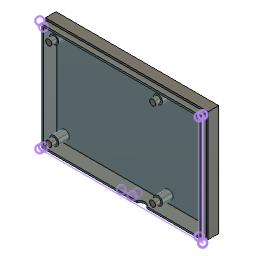
bottom-enclosure-v1 (Autodesk Fusion 360 design; units mm, degrees)
part number: 2026-06-12-23-29-13-626
Autodesk Fusion 360 part; units mm, degrees
note: some values were not read from the file. Set by a fixed rule: which sketch regions a step uses.
sketch "Sketch1" plane through (0, 0, 0) normal (0, 0, 1) x (1, 0, 0)
sketch "Sketch2" plane through (0, 0, 0) normal (0, 0, 1) x (1, 0, 0)
  line L0 (44.5, 30) -> (-44.5, 30)
  line L1 (-44.5, 30) -> (-44.5, -30)
  line L2 (-44.5, -30) -> (44.5, -30)
  line L3 (44.5, -30) -> (44.5, 30)
  line L4 (44.5, 30) -> (-44.5, -30) construction
  line L5 (-44.5, 30) -> (44.5, -30) construction
  dimension "d1" = 89
  dimension "d2" = 60
  constraint horizontal L0
  constraint perpendicular L0 L1
  constraint parallel L0 L2
  constraint parallel L1 L3
  constraint coincident L4 origin
  constraint coincident L5 origin
  measures "d1" distance of L1.end L2.end
  measures "d2" distance of L0.end L1.end
extrude "Extrude1" add sketch "Sketch2" along normal blind 1.5 makes body 1
sketch "Sketch3" plane through (0, 0, 1.5) normal (0, 0, 1) x (1, 0, 0)
  line L0 (44.5, -30) -> (44.5, 30)
  line L1 (44.5, 30) -> (-44.5, 30)
  line L2 (-44.5, 30) -> (-44.5, -30)
  line L3 (-44.5, -30) -> (44.5, -30)
  line L4 (42.5, 28) -> (-42.5, 28)
  line L5 (-42.5, 28) -> (-42.5, -28)
  line L6 (-42.5, -28) -> (42.5, -28)
  line L7 (42.5, -28) -> (42.5, 28)
  line L8 (42.5, 28) -> (-42.5, -28) construction
  line L9 (-42.5, 28) -> (42.5, -28) construction
  line L10 (44.5, 30) -> (-44.5, 30)
  line L11 (-44.5, 30) -> (-44.5, -30)
  line L12 (-44.5, -30) -> (44.5, -30)
  line L13 (44.5, -30) -> (44.5, 30)
  line L14 (44.5, 30) -> (-44.5, -30) construction
  line L15 (-44.5, 30) -> (44.5, -30) construction
  dimension "d5" = 85
  dimension "d6" = 56
  dimension "d7" = 89
  dimension "d8" = 60
  constraint horizontal L4
  constraint perpendicular L4 L5
  constraint parallel L4 L6
  constraint parallel L5 L7
  constraint coincident L8 origin
  constraint coincident L9 origin
  constraint horizontal L10
  constraint perpendicular L10 L11
  constraint parallel L10 L12
  constraint parallel L11 L13
  constraint coincident L14 origin
  constraint coincident L15 origin
  measures "d5" distance of L5.end L6.end
  measures "d6" distance of L4.end L5.end
  measures "d7" distance of L2.end L0.start
  measures "d8" distance of L1.end L2.end
extrude "Extrude2" add sketch "Sketch3" along normal blind 7.5 bodies 1
sketch "Sketch4" plane through (0, 0, 1.5) normal (0, 0, 1) x (1, 0, 0)
  line L0 (42.5, 28) -> (-42.5, 28)
  line L1 (-42.5, 28) -> (-42.5, -28)
  line L2 (-42.5, -28) -> (42.5, -28)
  line L3 (42.5, -28) -> (42.5, 28)
  circle A0 centre (-39, 24.5) radius 2.5
  circle A1 centre (-39, -24.5) radius 2.5
  circle A2 centre (19, 24.5) radius 2.5
  circle A3 centre (19, -24.5) radius 2.5
  dimension "d11" = 85
  dimension "d12" = 56
  dimension "d13" = 5
  dimension "d14" = 5
  dimension "d15" = 5
  dimension "d16" = 5
  dimension "d17" = 49
  dimension "d18" = 58
  dimension "d19" = 3.5
  dimension "d20" = 3.5
  constraint horizontal A0.centre A2.centre
  constraint horizontal A1.centre A3.centre
  constraint vertical A2.centre A3.centre
  measures "d11" distance of L1 L3
  measures "d12" distance of L0 L2
  measures "d13" diameter of A0
  measures "d14" diameter of A1
  measures "d15" diameter of A2
  measures "d16" diameter of A3
  measures "d17" distance of A0.centre A1.centre
  measures "d18" distance of A0.centre A2.centre
  measures "d19" distance of L0 A0.centre
  measures "d20" distance of L1 A1.centre
extrude "Extrude3" add sketch "Sketch4" along normal blind 6 contours A0 | A1 | A2 | A3 bodies 1
sketch "Sketch5" plane through (0, 0, 7.5) normal (0, 0, 1) x (1, 0, 0)
  circle A0 centre (-39, 24.5) radius 2.5
  circle A1 centre (-39, 24.5) radius 1.65
  circle A2 centre (-39, -24.5) radius 1.65
  circle A3 centre (19, -24.5) radius 1.65
  circle A4 centre (19, 24.5) radius 1.65
  dimension "d23" = 3.3
  dimension "d24" = 3.3
  dimension "d25" = 3.3
  dimension "d26" = 3.3
  constraint concentric A0 A1
  measures "d23" diameter of A1
  measures "d24" diameter of A2
  measures "d25" diameter of A3
  measures "d26" diameter of A4
extrude "Extrude4" add sketch "Sketch5" along normal blind 3 contours A1 | A2 | A3 | A4 bodies 1
sketch "Sketch6" plane through (0, 0, 1.5) normal (0, 0, 1) x (1, 0, 0)
  circle A0 centre (-39, -24.5) radius 2.5
  circle A1 centre (-39, 24.5) radius 2.5
  circle A2 centre (19, -24.5) radius 2.5
  circle A3 centre (19, 24.5) radius 2.5
  line L0 (42.5, 28) -> (-42.5, 28)
  line L1 (-42.5, 28) -> (-42.5, -28)
  line L2 (-42.5, -28) -> (42.5, -28)
  line L3 (42.5, -28) -> (42.5, 28)
sketch "Sketch7" plane through (0, 0, 9) normal (0, 0, 1) x (1, 0, 0)
  line L0 (42.5, 28) -> (42.5, -28)
  line L1 (42.5, -28) -> (-42.5, -28)
  line L2 (-42.5, -28) -> (-42.5, 28)
  line L3 (-42.5, 28) -> (42.5, 28)
  line L4 (44.5, -30) -> (44.5, 30)
  line L5 (44.5, 30) -> (-44.5, 30)
  line L6 (-44.5, 30) -> (-44.5, -30)
  line L7 (-44.5, -30) -> (44.5, -30)
  line L8 (0, 30) -> (5, 30)
  line L9 (5, 30) -> (5, 32)
  line L10 (5, 32) -> (0, 32)
  line L11 (0, 32) -> (0, 30)
  line L12 (0, 30) -> (-5, 30)
  line L13 (-5, 30) -> (-5, 32)
  line L14 (-5, 32) -> (0, 32)
  line L15 (0, 32) -> (0, 30)
  line L16 (0, -30) -> (5, -30)
  line L17 (5, -30) -> (5, -32)
  line L18 (5, -32) -> (0, -32)
  line L19 (0, -32) -> (0, -30)
  line L20 (0, -30) -> (-5, -30)
  line L21 (-5, -30) -> (-5, -32)
  line L22 (-5, -32) -> (0, -32)
  line L23 (0, -32) -> (0, -30)
  dimension "d29" = 5
  dimension "d30" = 2
  dimension "d31" = 2
  dimension "d32" = 5
  dimension "d33" = 2
  dimension "d34" = 5
  constraint horizontal L8
  constraint vertical L9
  constraint horizontal L10
  constraint vertical L11
  constraint midpoint L5 L8.start
  constraint horizontal L12
  constraint vertical L13
  constraint horizontal L14
  constraint vertical L15
  constraint horizontal L16
  constraint vertical L17
  constraint horizontal L18
  constraint vertical L19
  constraint midpoint L7 L16.start
  constraint horizontal L20
  constraint vertical L21
  constraint horizontal L22
  constraint vertical L23
  measures "d29" distance of L8.start L8.end
  measures "d30" distance of L8.start L10.end
  measures "d31" distance of L8.start L10.end
  measures "d32" distance of L16.start L16.end
  measures "d33" distance of L16.start L18.end
  measures "d34" distance of L16.start L20.end
extrude "Extrude5" add sketch "Sketch7" against normal blind 4 contours L7 L16 L17 L18 L19 L23 | L5 L8 L9 L10 L11 L15 | L7 L19 L20 L21 L22 L23 | L5 L11 L12 L13 L14 L15 bodies 1
extrude "Extrude6" add 2 faces at (-1.6667, -30.6667, 5) (-1.6667, 31.3333, 5) along direction (0, 0, -1) blind 4 on bodies 1 bodies 1
extrude "Extrude7" add 2 faces at (-1.6667, 31.3333, 1) (-1.6667, -30.6667, 1) along direction (0, 0, -1) blind 1 on bodies 1 bodies 1
sketch "Sketch8" plane through (0, 0, 9) normal (0, 0, 1) x (1, 0, 0)
  line L0 (42.5, 28) -> (42.5, -28)
  line L1 (42.5, -28) -> (-42.5, -28)
  line L2 (-42.5, -28) -> (-42.5, 28)
  line L3 (-42.5, 28) -> (42.5, 28)
  line L4 (44.5, -30) -> (44.5, 30)
  line L5 (44.5, 30) -> (5, 30)
  line L6 (5, 30) -> (5, 32)
  line L7 (5, 32) -> (-5, 32)
  line L8 (-5, 32) -> (-5, 30)
  line L9 (-5, 30) -> (-44.5, 30)
  line L10 (-44.5, 30) -> (-44.5, -30)
  line L11 (-44.5, -30) -> (-5, -30)
  line L12 (-5, -30) -> (-5, -32)
  line L13 (-5, -32) -> (5, -32)
  line L14 (5, -32) -> (5, -30)
  line L15 (5, -30) -> (44.5, -30)
  line L16 (5, -32) -> (-5, -32)
  line L17 (-5, -32) -> (-5, -30)
  line L18 (-5, -30) -> (5, -30)
  line L19 (5, -30) -> (5, -32)
  line L20 (5, 30) -> (-5, 30)
  line L21 (-5, 30) -> (-5, 32)
  line L22 (-5, 32) -> (5, 32)
  line L23 (5, 32) -> (5, 30)
  constraint horizontal L16
  constraint vertical L17
  constraint horizontal L18
  constraint vertical L19
  constraint coincident L11.end L12.start
  constraint coincident L13.end L14.start
  constraint horizontal L20
  constraint vertical L21
  constraint horizontal L22
  constraint vertical L23
  constraint coincident L7.end L8.start
  constraint coincident L5.end L6.start
extrude "Extrude8" cut sketch "Sketch8" against normal blind 2 contours L12 L13 L14 L16 L17 L18 L19 | L6 L7 L8 L20 L21 L22 L23 bodies 1
fillet "Fillet1" radius 1 1 edges at (0, 32, 7) on bodies 1
fillet "Fillet2" radius 1 1 edges at (0, -32, 7) on bodies 1
extrude "Extrude9" cut 1 faces at (14.1667, 28, 4) along direction (0, 1, 0) blind 1 on bodies 1 bodies 1
extrude "Extrude10" cut 1 faces at (42.5, -9, 4) along direction (1, 0, 0) blind 1 on bodies 1 bodies 1
extrude "Extrude11" cut 1 faces at (-13.8333, -28, 4) along direction (0, -1, 0) blind 1 on bodies 1 bodies 1
extrude "Extrude12" cut 1 faces at (-42.5, 9.6667, 6.5) along direction (-1, 0, 0) blind 1 on bodies 1 bodies 1
extrude "Extrude13" add 1 faces at (44.5, -10, 6) along direction (1, 0, 0) blind 1 on bodies 1 bodies 1
extrude "Extrude14" add 1 faces at (-44.5, 10, 6) along direction (-1, 0, 0) blind 1 on bodies 1 bodies 1
extrude "Extrude15" add 1 faces at (-32, 30, 5.3333) along direction (0, 1, 0) blind 1 on bodies 1 bodies 1
extrude "Extrude16" add 1 faces at (-32, -30, 5.3333) along direction (0, -1, 0) blind 1 on bodies 1 bodies 1
sketch "Sketch9" plane through (0, 0, 0) normal (0, 0, -1) x (-1, 0, 0)
  line L0 (-5, -31) -> (-5, -32)
  line L1 (-5, -32) -> (5, -32)
  line L2 (5, -32) -> (5, -31)
  line L3 (5, -31) -> (45.5, -31)
  line L4 (45.5, -31) -> (45.5, 31)
  line L5 (45.5, 31) -> (5, 31)
  line L6 (5, 31) -> (5, 32)
  line L7 (5, 32) -> (-5, 32)
  line L8 (-5, 32) -> (-5, 31)
  line L9 (-5, 31) -> (-45.5, 31)
  line L10 (-45.5, 31) -> (-45.5, -31)
  line L11 (-45.5, -31) -> (-5, -31)
  line L12 (-5, 32) -> (5, 32)
  line L13 (5, 32) -> (5, 31)
  line L14 (5, 31) -> (-5, 31)
  line L15 (-5, 31) -> (-5, 32)
  constraint horizontal L12
  constraint vertical L13
  constraint horizontal L14
  constraint vertical L15
  constraint coincident L5.end L6.start
  constraint coincident L7.end L8.start
extrude "Extrude17" cut sketch "Sketch9" against normal blind 20 contours L6 L7 L8 L12 L13 L14 L15 bodies 1
sketch "Sketch10" plane through (0, 0, 0) normal (0, 0, -1) x (-1, 0, 0)
  line L0 (45.5, 31) -> (-45.5, 31)
  line L1 (-45.5, 31) -> (-45.5, -31)
  line L2 (-45.5, -31) -> (-5, -31)
  line L3 (-5, -31) -> (-5, -32)
  line L4 (-5, -32) -> (5, -32)
  line L5 (5, -32) -> (5, -31)
  line L6 (5, -31) -> (45.5, -31)
  line L7 (45.5, -31) -> (45.5, 31)
  line L8 (-5, -31) -> (5, -31)
  line L9 (5, -31) -> (5, -32)
  line L10 (5, -32) -> (-5, -32)
  line L11 (-5, -32) -> (-5, -31)
  constraint horizontal L8
  constraint vertical L9
  constraint horizontal L10
  constraint vertical L11
  constraint coincident L4.end L5.start
  constraint coincident L2.end L3.start
extrude "Extrude18" cut sketch "Sketch10" against normal blind 20 contours L3 L4 L5 L8 L9 L10 L11 bodies 1
sketch "Sketch11" plane through (0, -31, 0) normal (0, -1, 0) x (1, 0, 0)
  line L0 (-45.5, 0) -> (45.5, 0)
  line L1 (45.5, 0) -> (45.5, 9)
  line L2 (45.5, 9) -> (-45.5, 9)
  line L3 (-45.5, 9) -> (-45.5, 0)
  line L4 (3, 6) -> (-3, 6)
  line L5 (-3, 6) -> (-3, 3)
  line L6 (-3, 3) -> (3, 3)
  line L7 (3, 3) -> (3, 6)
  line L8 (3, 6) -> (-3, 3) construction
  line L9 (-3, 6) -> (3, 3) construction
  point P0 (0, 4.5)
  dimension "d67" = 9
  dimension "d68" = 6
  dimension "d69" = 3
  dimension "d70" = 4.5
  constraint horizontal L4
  constraint perpendicular L4 L5
  constraint parallel L4 L6
  constraint parallel L5 L7
  constraint coincident L8 P0
  constraint coincident L9 P0
  measures "d67" distance of L0 L2
  measures "d68" distance of L5.end L6.end
  measures "d69" distance of L4.end L5.end
  measures "d70" distance of origin P0
extrude "Extrude19" cut sketch "Sketch11" against normal blind 1.5 contours L4 L5 L6 L7 bodies 1
sketch "Sketch12" plane through (0, 0, 9) normal (0, 0, 1) x (1, 0, 0)
  line L0 (43.5, -29) -> (-43.5, -29)
  line L1 (-43.5, -29) -> (-43.5, 29)
  line L2 (-43.5, 29) -> (43.5, 29)
  line L3 (43.5, 29) -> (43.5, -29)
  line L4 (45.5, -31) -> (45.5, 31)
  line L5 (45.5, 31) -> (-45.5, 31)
  line L6 (-45.5, 31) -> (-45.5, -31)
  line L7 (-45.5, -31) -> (45.5, -31)
  dimension "d73" = 2
  measures "d73" distance of L0 L7
sketch "Sketch13" plane through (0, 31, 0) normal (0, 1, 0) x (-1, 0, 0)
  line L0 (-45.5, 0) -> (45.5, 0)
  line L1 (45.5, 0) -> (45.5, 9)
  line L2 (45.5, 9) -> (-45.5, 9)
  line L3 (-45.5, 9) -> (-45.5, 0)
  line L4 (3, 6) -> (-3, 6)
  line L5 (-3, 6) -> (-3, 3)
  line L6 (-3, 3) -> (3, 3)
  line L7 (3, 3) -> (3, 6)
  line L8 (3, 6) -> (-3, 3) construction
  line L9 (-3, 6) -> (3, 3) construction
  point P0 (0, 4.5)
  dimension "d74" = 6
  dimension "d75" = 3
  dimension "d76" = 4.5
  constraint horizontal L4
  constraint perpendicular L4 L5
  constraint parallel L4 L6
  constraint parallel L5 L7
  constraint coincident L8 P0
  constraint coincident L9 P0
  measures "d74" distance of L5.end L6.end
  measures "d75" distance of L4.end L5.end
  measures "d76" distance of L0 P0
extrude "Extrude20" cut sketch "Sketch13" against normal blind 1.5 contours L4 L5 L6 L7 bodies 1
sketch "Sketch14" plane through (0, 0, 9) normal (0, 0, 1) x (1, 0, 0)
  point P0 (45.5, -31)
  point P1 (-45.5, -31)
  point P2 (-45.5, 31)
  dimension "d79" = 91
  dimension "d80" = 62
  measures "d79" distance of P0 P1
  measures "d80" distance of P1 P2
sketch "Sketch15" plane through (0, 0, 9) normal (0, 0, 1) x (1, 0, 0)
  point P0 (-43.5, -29)
  point P1 (43.5, -29)
  dimension "d81" = 87
  measures "d81" distance of P0 P1
sketch "Sketch16" plane through (0, -31, 0) normal (0, -1, 0) x (1, 0, 0)
  line L0 (-3, 6) -> (3, 6)
  line L1 (3, 6) -> (3, 3)
  line L2 (3, 3) -> (-3, 3)
  line L3 (-3, 3) -> (-3, 6)
  line L4 (-45.5, 0) -> (45.5, 0)
  line L5 (45.5, 0) -> (45.5, 9)
  line L6 (45.5, 9) -> (-45.5, 9)
  line L7 (-45.5, 9) -> (-45.5, 0)
  circle A0 centre (11.5, 10.2501) radius 3
  point P0 (-43.5, 9)
  point P1 (43.5, 9)
  dimension "d82" = 87
  dimension "d83" = 6
  dimension "d84" = 32
  measures "d82" distance of P0 P1
  measures "d83" diameter of A0
  measures "d84" horizontal distance of P1 A0.centre
extrude "Extrude21" cut sketch "Sketch16" against normal blind 5 contours L6 A0 picked at (11.9149, 8.5068) bodies 1
sketch "Sketch17" plane through (0, 0, 9) normal (0, 0, 1) x (1, 0, 0)
  line L0 (43.5, 29) -> (43.5, -29)
  line L1 (45.5, -31) -> (45.5, 31)
  point P0 (-45.5, 31)
  point P1 (45.5, 31)
  point P2 (45.5, -31)
  point P3 (-43.5, 29)
  point P4 (-43.5, -29)
  dimension "d87" = 91
  dimension "d88" = 62
  dimension "d89" = 2
  dimension "d90" = 87
  dimension "d91" = 58
  measures "d87" distance of P0 L1.end
  measures "d88" distance of P1 L1.start
  measures "d89" distance of L0 L1
  measures "d90" distance of L0.start P3
  measures "d91" distance of P3 P4
sketch "Sketch18" plane through (0, -31, 0) normal (0, -1, 0) x (1, 0, 0)
  arc A0 (8.7729, 9) -> (14.2271, 9) centre (11.5, 10.2501) ccw
  line L0 (8.7729, 9) -> (-45.5, 9)
  line L1 (-45.5, 9) -> (-45.5, 0)
  line L2 (-45.5, 0) -> (45.5, 0)
  line L3 (45.5, 0) -> (45.5, 9)
  line L4 (45.5, 9) -> (14.2271, 9)
  line L5 (-3, 6) -> (3, 6)
  line L6 (3, 6) -> (3, 3)
  line L7 (3, 3) -> (-3, 3)
  line L8 (-3, 3) -> (-3, 6)
sketch "Sketch19" plane through (0, -31, 0) normal (0, -1, 0) x (1, 0, 0)
  line L0 (-45.5, 9) -> (45.5, 9)
  line L1 (-3, 6) -> (3, 6)
  point P0 (-3, 6)
  point P1 (3, 6)
  point P2 (3, 3)
  dimension "d92" = 6
  dimension "d93" = 3
  dimension "d94" = 3
  measures "d92" distance of P0 L1.end
  measures "d93" distance of L0 L1
  measures "d94" distance of P1 P2
extrude "Extrude22" add sketch "Sketch18" along normal blind 1.5 separate body contours L5 L6 L7 L8 makes body 2
extrude "Extrude23" cut 1 faces at (-1, -32.5, 5) along direction (0, 1, 0) blind 1 on bodies 2 bodies 2
extrude "Extrude24" cut 1 faces at (-1, -31.5, 5) along direction (0, 1, 0) blind 0.5 on bodies 2 bodies 2
extrude "Extrude25" add 1 faces at (-1, -29.5, 5) along direction (0, -1, 0) blind 1 on bodies 1 bodies 1 2
extrude "Extrude26" add 1 faces at (-1, -30.5, 5) along direction (0, -1, 0) blind 0.5 on bodies 1 bodies 1
extrude "Extrude27" add 1 faces at (1, 29.5, 5) along direction (0, 1, 0) blind 1.5 on bodies 1 bodies 1
sketch "Sketch20" plane through (0, 0, 9) normal (0, 0, 1) x (1, 0, 0)
  line L0 (-44.5, 30) -> (44.5, 30)
  line L1 (44.5, 30) -> (44.5, -30)
  line L2 (44.5, -30) -> (-44.5, -30)
  line L3 (-44.5, -30) -> (-44.5, 30)
  line L4 (-45.5, 31) -> (45.5, 31)
  line L5 (45.5, 31) -> (45.5, -31)
  line L6 (45.5, -31) -> (-45.5, -31)
  line L7 (-45.5, -31) -> (-45.5, 31)
  constraint horizontal L0
  constraint vertical L1
  constraint horizontal L2
  constraint vertical L3
  constraint horizontal L4
  constraint vertical L5
  constraint horizontal L6
  constraint vertical L7
extrude "Extrude28" cut sketch "Sketch20" against normal blind 3 bodies 1
